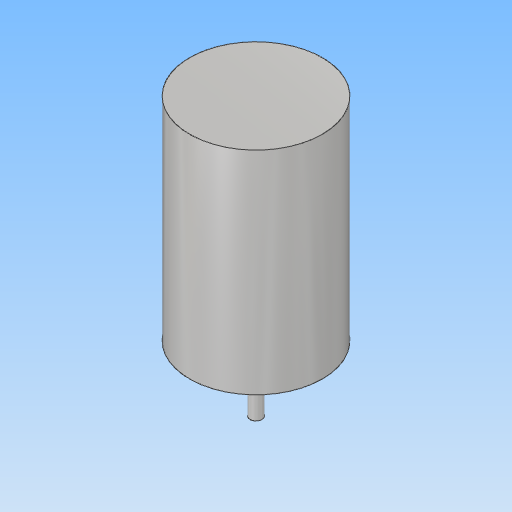
# Autodesk Inventor part: 540DCMotor
Saved by Autodesk Inventor 2017 (Build 210142000, 142)
## iProperties
Created: 2016-10-13
Part Number: 540DCMotor
Material: Generic
Document SubType Name: Modeling
Designer: techn
Density: 1 g/cm^3
Appearance: Aluminum - Polished
Author: techn
Autodesk Inventor part; units mm, degrees
ref_plane "YZ Plane" through (0, 0, 0) normal (1, 0, 0) x (0, 1, 0)
ref_plane "XZ Plane" through (0, 0, 0) normal (0, 1, 0) x (-1, 0, 0)
ref_plane "XY Plane" through (0, 0, 0) normal (0, 0, 1) x (1, 0, 0)
sketch "Sketch1" plane through (0, 0, 0) normal (0, 0, 1) x (1, 0, 0)
  line L0 (0, 0) -> (1.6, 0)
  line L1 (1.6, 0) -> (1.6, 12.446)
  line L2 (0, 17.2085) -> (17.5, 17.2085)
  line L3 (0, 12.446) -> (6.5, 12.446)
  line L4 (6.5, 12.446) -> (6.5, 17.2085)
  line L5 (17.5, 17.2085) -> (17.5, 73.0885)
  line L6 (17.5, 73.0885) -> (0, 73.0885)
  line L7 (0, 73.0885) -> (0, 0)
  dimension "d0" = 1.6
  dimension "d1" = 12.446
  dimension "d2" = 17.5
  dimension "d3" = 6.5
  dimension "d4" = 4.7625
  dimension "d5" = 55.88
  constraints: 16 end point, 4 point on line, 3 horizontal, 2 perpendicular, 2 vertical, 1 parallel
  measures "d0" distance of L0.start L0.end
  measures "d1" distance of L0.end L1.end
  measures "d2" distance of L2.start L2.end
  measures "d3" distance of L3.start L3.end
  measures "d4" distance of L3.end L4.end
  measures "d5" distance of L2.end L5.end
revolve "Revolution1" add sketch "Sketch1" angle 360 about axis through (0, 73.0885, 0) along (0, -1, 0)
sketch "Sketch2" plane through (0, 17.2085, 0) normal (0, -1, 0) x (1, 0, 0)
  circle A0 centre (0, 0) radius 12.5
  circle A1 centre (-12.5, 0) radius 1.6
  circle A2 centre (12.5, 0) radius 1.6
  point P0 (0, 0)
  dimension "d7" = 25
  dimension "d8" = 3.2
  dimension "d9" = 3.2
  constraints: 3 centre point, 2 point on circle, 1 coincident
  measures "d7" diameter of A0
  measures "d8" diameter of A1
  measures "d9" diameter of A2
extrude "Extrusion1" cut sketch "Sketch2" against normal blind 6.35 contours A0 A2 | A0 A2 | A1 A0 | A0 A1
body "Solid1"
